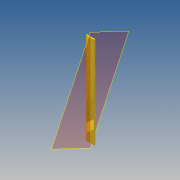
# Autodesk Inventor part: Version 2 field plate
Saved by Autodesk Inventor 2011 SP1 (Build 150282100, 282)
## iProperties
Created: 2006-06-02
Part Number: Version 2 field plate
Document SubType Name: Modeling
Designer: Jon
Density: 1 g/cm^3
Author: Jon
Autodesk Inventor part; units mm, degrees
ref_plane "YZ Plane" through (0, 0, 0) normal (1, 0, 0) x (0, 1, 0)
ref_plane "XZ Plane" through (0, 0, 0) normal (0, 1, 0) x (-1, 0, 0)
ref_plane "XY Plane" through (0, 0, 0) normal (0, 0, 1) x (1, 0, 0)
sketch "Sketch1" plane through (0, 0, 0) normal (0, 0, 1) x (1, 0, 0)
  line L0 (2.4705, -2.1641) -> (-67.5295, -2.1641)
  line L1 (-67.5295, -2.1641) -> (-67.5295, 10.5359)
  line L2 (-67.5295, 10.5359) -> (2.4705, 10.5359)
  line L3 (2.4705, 10.5359) -> (2.4705, -2.1641)
  dimension "d0" = 12.7
  dimension "d1" = 70
  constraints: 8 end point, 2 parallel, 1 horizontal, 1 perpendicular
  measures "d0" distance of L0.end L1.end
  measures "d1" distance of L1.end L2.end
extrude "Extrusion1" add sketch "Sketch1" along normal blind 567.2
sketch "Sketch2" plane through (2.4705, -2.1641, 0) normal (1, 0, 0) x (0, 0, -1)
  line L0 (-567.3829, 6.35) -> (0, 6.35) construction
  line L1 (0, 12.7) -> (-567.2, 12.7) construction
  line L2 (-567.2, 12.7) -> (-567.2, 0) construction
  point P0 (-543.6, 6.35)
  point P1 (-33.6, 6.35)
  point P2 (-133.6, 6.35)
  point P3 (-238.6, 6.35)
  point P4 (-338.6, 6.35)
  point P5 (-443.6, 6.35)
  dimension "d4" = 6.35
  dimension "d5" = 23.6
  dimension "d6" = 100
  dimension "d7" = 105
  dimension "d8" = 100
  dimension "d9" = 105
  dimension "d10" = 100
  dimension "d11" = 33.6
  dimension "d12" = 567.3829
  constraints: 6 point on line, 2 end point, 1 horizontal
  measures "d4" distance from line of L1 L0.start
  measures "d5" distance from line of point (-543.6, 6.35) L2
  measures "d6" distance of point (-443.6, 6.35) point (-543.6, 6.35)
  measures "d7" distance of point (-338.6, 6.35) point (-443.6, 6.35)
  measures "d8" distance of point (-238.6, 6.35) point (-338.6, 6.35)
  measures "d9" distance of point (-133.6, 6.35) point (-238.6, 6.35)
  measures "d10" distance of point (-33.6, 6.35) point (-133.6, 6.35)
  measures "d11" distance of point (-33.6, 6.35) L0.end
  measures "d12" distance of L0.start L0.end
hole "Hole1" [suppressed]
sketch "Sketch3" plane through (0, 0, 567.2) normal (0, 0, 1) x (1, 0, 0)
  line L0 (-67.5295, -2.1641) -> (-67.5295, 10.5359) projected
  line L1 (-67.5295, 10.5359) -> (2.4705, 10.5359) projected
  line L2 (2.4705, -2.1641) -> (-67.5295, -2.1641) projected
  line L3 (2.4705, 10.5359) -> (2.4705, -2.1641) projected
extrude "Extrusion2" add sketch "Sketch3" along normal blind 150
sketch "Sketch4" plane through (0, 0, 0) normal (0, 0, -1) x (-1, 0, 0)
  line L0 (-2.4705, -2.1641) -> (67.5295, -2.1641) projected
  line L1 (67.5295, -2.1641) -> (67.5295, 10.5359) projected
  line L2 (67.5295, 10.5359) -> (-2.4705, 10.5359) projected
  line L3 (-2.4705, 10.5359) -> (-2.4705, -2.1641) projected
extrude "Extrusion3" add sketch "Sketch4" along normal blind 150
sketch "Sketch5" plane through (2.4705, -2.1641, 717.2) normal (1, 0, 0) x (0, 0, -1)
  circle A0 centre (73.972, 6.35) radius 3.9687 projected
  circle A1 centre (113.972, 6.35) radius 3.9687 projected
  circle A2 centre (748.257, 6.35) radius 3.9687 projected
  circle A3 centre (798.257, 6.35) radius 3.9687 projected
hole "Hole2" [suppressed]
sketch "Sketch6" plane through (2.4705, -2.1641, 717.2) normal (1, 0, 0) x (0, 0, -1)
  line L0 (867.2, 0) -> (0, 0) projected
  line L1 (0, 12.7) -> (0, 0) projected
  line L2 (0, 12.7) -> (867.2, 12.7) projected
  line L3 (63.972, 12.7) -> (63.972, 0)
  line L4 (63.972, 12.7) -> (0, 12.7)
  line L5 (0, 0) -> (63.972, 0)
  line L6 (0, 0) -> (0, 12.7)
  circle A0 centre (73.972, 6.35) radius 3.9687 projected
  dimension "d31" = 10
  constraints: 8 end point, 3 perpendicular, 2 point on line, 1 collinear
  measures "d31" distance from line of L3 A0.centre
extrude "Extrusion4" cut sketch "Sketch6" against normal blind 70 contours L0 L1 L2 L3
sketch "Sketch7" plane through (2.4705, -2.1641, 653.228) normal (1, 0, 0) x (0, 0, -1)
  line L0 (803.228, 0) -> (0, 0) projected
  line L1 (0, 12.7) -> (803.228, 12.7) projected
  line L2 (803.228, 0) -> (803.228, 12.7) projected
  circle A0 centre (734.285, 6.35) radius 3.9687 projected
  line L3 (749.285, 12.7) -> (749.285, 0)
  line L4 (749.285, 0) -> (803.228, 0)
  line L5 (803.228, 1.1687) -> (803.228, 12.7)
  line L6 (803.228, 12.7) -> (749.285, 12.7)
  dimension "d34" = 15
  constraints: 8 end point, 3 point on line, 2 collinear, 2 perpendicular
  measures "d34" distance from line of L3 A0.centre
extrude "Extrusion5" cut sketch "Sketch7" against normal blind 70 contours L0 L3 L1 L2
fillet "Fillet1" radius 3 4 edges at (2.4705, -2.1641, 278.5855) (-32.5295, -2.1641, -96.057) (-67.5295, -2.1641, 278.5855) (-32.5295, -2.1641, 653.228)
fillet "Fillet2" radius 9 4 edges at (-32.5295, 10.5359, 653.228) (-67.5295, 10.5359, 278.5855) (-32.5295, 10.5359, -96.057) (2.4705, 10.5359, 278.5855)
sketch "Sketch8" plane through (-67.5295, 0.8359, 238.6) normal (-1, 0, 0) x (0, 0, 1)
  line L0 (38.016, -32.096) -> (38.016, 13.904) projected
  line L1 (405.628, 9.7) -> (-325.657, 9.7) projected
  line L2 (38.016, 3.35) -> (67.7675, 3.35) construction
  line L3 (49.521, 11.9848) -> (49.521, 0.9719) construction
  point P0 (49.521, 3.35)
  dimension "d39" = 11.505
  dimension "d40" = 6.35
  constraints: 4 end point, 3 point on line, 1 parallel, 1 perpendicular
  measures "d39" distance between parallel lines of L3 L0
  measures "d40" distance between parallel lines of L1 L2
hole "Hole3" [suppressed]
sketch "Sketch9" plane through (2.4705, 0.8359, 338.6) normal (1, 0, 0) x (0, 0, -1)
  arc A0 (49.011, 3.658) -> (51.947, 3.658) centre (50.479, 3.35) ccw projected
  constraints: 1 coincident
hole "Hole4" [suppressed]
ref_plane "Work Plane1" through (-32.5295, -2.1641, 650.228) normal (-1, 0, 0) x (0, 0.9041723, -0.427168)
body "Solid1"
